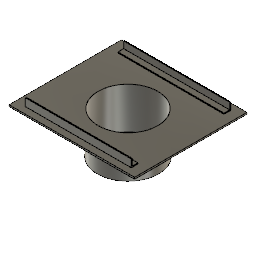
protec_tubage_2 v3 (Autodesk Fusion 360 design; units mm, degrees)
Autodesk Fusion 360 part; units mm, degrees
sketch "Esquisse1" plane through (0, 0, 0) normal (0, 0, 1) x (1, 0, 0)
  line L0 (190, -170) -> (-190, -170)
  line L1 (-190, -170) -> (-190, 170)
  line L2 (-190, 170) -> (190, 170)
  line L3 (190, 170) -> (190, -170)
  line L4 (190, -170) -> (-190, 170) construction
  line L5 (-190, -170) -> (190, 170) construction
  dimension "d1" = 380
  dimension "d2" = 340
  constraint horizontal L0
  constraint perpendicular L0 L1
  constraint parallel L0 L2
  constraint parallel L1 L3
  constraint coincident L4 origin
  constraint coincident L5 origin
  measures "d1" distance of L1.end L2.end
  measures "d2" distance of L0.start L2.end
extrude "Extrusion1" add sketch "Esquisse1" along normal blind 5 makes body 1
sketch "Esquisse2" plane through (0, 0, 0) normal (0, 0, -1) x (1, 0, 0)
  line L0 (-190, -170) -> (190, -170)
  line L1 (190, -170) -> (190, 170)
  line L2 (190, 170) -> (-190, 170)
  line L3 (-190, 170) -> (-190, -170)
  circle A0 centre (0, 0) radius 93
  dimension "d5" = 186
  constraint coincident A0.centre origin
  measures "d5" diameter of A0
extrude "Extrusion2" add sketch "Esquisse2" along normal blind 120 contours A0 bodies 1
sketch "Esquisse3" plane through (0, 0, -120) normal (0, 0, -1) x (1, 0, 0)
  circle A0 centre (0, 0) radius 93
  circle A1 centre (0, 0) radius 90
  dimension "d8" = 180
  constraint coincident A0.centre A1.centre
  measures "d8" diameter of A1
extrude "Extrusion3" cut sketch "Esquisse3" against normal blind 125 contours A1 bodies 1
sketch "Esquisse4" plane through (0, 0, 5) normal (0, 0, 1) x (-1, 0, 0)
  circle A0 centre (0, 0) radius 90
  line L0 (-190, -170) -> (190, -170)
  line L1 (190, -170) -> (190, 170)
  line L2 (190, 170) -> (-190, 170)
  line L3 (-190, 170) -> (-190, -170)
  line L4 (160.0001, -149.9995) -> (-159.9999, -149.9995)
  line L5 (-159.9999, -149.9995) -> (-159.9999, -129.9995)
  line L6 (-159.9999, -129.9995) -> (160.0001, -129.9995)
  line L7 (160.0001, -129.9995) -> (160.0001, -149.9995)
  dimension "d11" = 320
  dimension "d12" = 20
  constraint horizontal L4
  constraint vertical L5
  constraint horizontal L6
  constraint vertical L7
  measures "d11" distance of L4.start L4.end
  measures "d12" distance of L4.start L6.end
extrude "Extrusion4" add sketch "Esquisse4" along normal blind 3 separate body contours L4 L5 L6 L7 makes body 2
sketch "Esquisse11" plane through (0, 0, 8) normal (0, 0, 1) x (-1, 0, 0)
  line L0 (160.0001, -129.9995) -> (-159.9999, -129.9995)
  line L1 (-159.9999, -129.9995) -> (-159.9999, -149.9995)
  line L2 (-159.9999, -149.9995) -> (160.0001, -149.9995)
  line L3 (160.0001, -149.9995) -> (160.0001, -129.9995)
  line L4 (160.0001, -149.9995) -> (-159.9999, -149.9995)
  line L5 (-159.9999, -149.9995) -> (-159.9999, -146.9995)
  line L6 (-159.9999, -146.9995) -> (160.0001, -146.9995)
  line L7 (160.0001, -146.9995) -> (160.0001, -149.9995)
  dimension "d16" = 320
  dimension "d17" = 3
  constraint horizontal L4
  constraint vertical L5
  constraint horizontal L6
  constraint vertical L7
  constraint coincident L2.end L3.start
  measures "d16" distance of L2.end L1.end
  measures "d17" distance of L2.end L6.end
extrude "Extrusion5" add sketch "Esquisse11" along normal blind 20 contours L1 L2 L3 L4 L5 L6 L7 bodies 2
sketch "Esquisse12" plane through (0, 0, 5) normal (0, 0, 1) x (-1, 0, 0)
  circle A0 centre (0, 0) radius 90
  line L0 (-190, -170) -> (190, -170)
  line L1 (190, -170) -> (190, 170)
  line L2 (190, 170) -> (-190, 170)
  line L3 (-190, 170) -> (-190, -170)
  line L4 (-159.9999, 129.9997) -> (160.0001, 129.9997)
  line L5 (160.0001, 129.9997) -> (160.0001, 149.9997)
  line L6 (160.0001, 149.9997) -> (-159.9999, 149.9997)
  line L7 (-159.9999, 149.9997) -> (-159.9999, 129.9997)
  dimension "d20" = 320
  dimension "d21" = 20
  constraint horizontal L4
  constraint vertical L5
  constraint horizontal L6
  constraint vertical L7
  measures "d20" distance of L4.start L4.end
  measures "d21" distance of L4.start L6.end
extrude "Extrusion6" add sketch "Esquisse12" along normal blind 3 contours L4 L5 L6 L7 bodies 1
sketch "Esquisse13" plane through (0, 0, 8) normal (0, 0, 1) x (-1, 0, 0)
  line L0 (-159.9999, 149.9997) -> (-159.9999, 129.9997)
  line L1 (-159.9999, 129.9997) -> (160.0001, 129.9997)
  line L2 (160.0001, 129.9997) -> (160.0001, 149.9997)
  line L3 (160.0001, 149.9997) -> (-159.9999, 149.9997)
  line L4 (-159.9999, 149.9997) -> (160.0001, 149.9997)
  line L5 (160.0001, 149.9997) -> (160.0001, 146.9997)
  line L6 (160.0001, 146.9997) -> (-159.9999, 146.9997)
  line L7 (-159.9999, 146.9997) -> (-159.9999, 149.9997)
  dimension "d24" = 320
  dimension "d25" = 3
  constraint horizontal L4
  constraint vertical L5
  constraint horizontal L6
  constraint vertical L7
  constraint coincident L0.start L3.end
  measures "d24" distance of L0.start L2.end
  measures "d25" distance of L0.start L6.end
extrude "Extrusion7" add sketch "Esquisse13" along normal blind 20 contours L0 L2 L3 L4 L5 L6 L7 bodies 1
